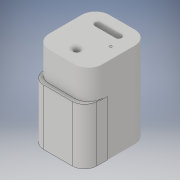
# Autodesk Inventor part: pencil sharpener
Saved by Autodesk Inventor 2017 (Build 210142000, 142)
## iProperties
Created: 2018-03-27
Part Number: pencil sharpener
Material: Generic
Document SubType Name: Modeling
Designer: Braxton
Density: 1 g/cm^3
Appearance: Default
Author: Braxton
Autodesk Inventor part; units mm, degrees
ref_plane "YZ Plane" through (0, 0, 0) normal (1, 0, 0) x (0, 1, 0)
ref_plane "XZ Plane" through (0, 0, 0) normal (0, 1, 0) x (-1, 0, 0)
ref_plane "XY Plane" through (0, 0, 0) normal (0, 0, 1) x (1, 0, 0)
sketch "Sketch1" plane through (0, 0, 0) normal (0, 1, 0) x (-1, 0, 0)
  line L0 (4.0465, 0) -> (4.0465, -4.1391)
  line L1 (1.9447, -6.241) -> (0, -6.241)
  arc A0 (1.9447, -6.241) -> (4.0465, -4.1391) centre (1.9447, -4.1391) ccw
  line L2 (4.0465, 0) -> (0, 0)
  line L3 (0, 0) -> (0, -6.241) construction
  line L4 (-4.0465, 0) -> (-4.0465, -4.1391)
  line L5 (-1.9447, -6.241) -> (0, -6.241)
  arc A1 (-4.0465, -4.1391) -> (-1.9447, -6.241) centre (-1.9447, -4.1391) ccw
  line L6 (-4.0465, 0) -> (0, 0)
  line L7 (0, 0) -> (0, 2.7914) construction
  dimension "d9" = 6.241
  dimension "d11" = 4.0465
  dimension "d12" = 2.1019
  constraints: 16 end point, 4 point on circle, 3 symmetric about line, 2 centre point, 2 collinear, 2 horizontal, 2 perpendicular, 2 tangent, 2 vertical, 1 other
  measures "d9" distance between parallel lines of L2 L1
  measures "d11" distance between parallel lines of L0 L3
  measures "d12" radius of A0
extrude "bace bottom" add sketch "Sketch1" along normal blind 7.3163
sketch "Sketch3" plane through (0, 7.3163, 0) normal (0, 1, 0) x (1, 0, 0)
  line L0 (1.9447, 6.241) -> (-1.9447, 6.241) projected
  line L1 (0, 6.241) -> (0, -3.1186) construction
  line L2 (0, 6.241) -> (-1.9447, 6.241)
  arc A0 (-1.9447, 6.241) -> (-4.0465, 4.1391) centre (-1.9447, 4.1391) ccw projected
  line L3 (-4.0465, 4.1391) -> (-4.0465, -0.825)
  line L4 (-1.9447, -2.9269) -> (0, -2.9269)
  arc A1 (-4.0465, -0.825) -> (-1.9447, -2.9269) centre (-1.9447, -0.825) ccw
  arc A2 (-1.9447, 6.241) -> (-4.0465, 4.1391) centre (-1.9447, 4.1391) ccw
  line L5 (0, 6.241) -> (1.9447, 6.241)
  arc A3 (4.0465, 4.1391) -> (1.9447, 6.241) centre (1.9447, 4.1391) ccw
  line L6 (4.0465, 4.1391) -> (4.0465, -0.825)
  line L7 (1.9447, -2.9269) -> (0, -2.9269)
  arc A4 (1.9447, -2.9269) -> (4.0465, -0.825) centre (1.9447, -0.825) ccw
  constraints: 14 end point, 8 point on circle, 5 symmetric about line, 5 tangent, 4 centre point, 2 vertical, 1 equal radius, 1 horizontal, 1 midpoint, 1 perpendicular, 1 point on line, 2 other
extrude "sharpener top" add sketch "Sketch3" along normal blind 4.6207
sketch "Sketch6" plane through (0, 0, 0) normal (1, 0, 0) x (0, 1, 0)
  line L0 (11.9369, 0.825) -> (11.9369, 2.9269) projected
  arc A0 (11.2464, 0.9441) -> (11.9369, 1.6347) centre (11.2464, 1.6347) ccw
  arc A1 (11.9369, -0.3815) -> (11.2464, 0.3091) centre (11.2464, -0.3815) ccw construction
  line L1 (11.9369, -4.1391) -> (11.9369, 0.825) projected
  line L2 (11.2464, 0.6266) -> (11.9369, 0.6266)
  line L3 (11.2464, 0.9441) -> (11.2464, 0.6266)
  line L4 (11.2464, 0.3091) -> (11.2464, 0.6266) construction
  line L5 (11.9369, 1.6347) -> (11.9369, 0.6266)
  line L6 (7.3163, 2.9269) -> (11.9369, 2.9269) projected
  point P0 (0, 0)
  dimension "d34" = 1.2922
  dimension "d37" = 2.0161
  constraints: 8 end point, 4 point on circle, 3 collinear, 3 point on line, 3 tangent, 2 centre point, 2 line through centre, 1 equal radius, 1 perpendicular, 1 vertical
  measures "d34" distance from line of L5.start L6
  measures "d37" distance of A1.start L5.start
revolve "sharpener hole" cut sketch "Sketch6" angle 360 about axis through (0, 11.2464, 0.6266) along (0, 1, 0)
sketch "Sketch7" plane through (0, 11.2464, 0.6266) normal (0, 1, 0) x (1, 0, 0)
  circle A0 centre (0, 0) radius 0.3175 projected
  circle A1 centre (0, 0) radius 0.3897
  point P0 (0, 0.6266)
  constraints: 1 centre point, 1 coincident
extrude "Extrusion of sharpener hole" cut sketch "Sketch7" against normal blind 1.5875 contours A0
sketch "Sketch8" plane through (0, 11.9369, 0) normal (0, 1, 0) x (1, 0, 0)
  line L0 (-1.5785, 4.1397) -> (1.5785, 4.1397) construction
  line L1 (-1.5785, 3.6661) -> (1.5785, 3.6661)
  line L2 (1.5785, 4.6133) -> (-1.5785, 4.6133)
  arc A0 (-1.5785, 4.6133) -> (-1.5785, 3.6661) centre (-1.5785, 4.1397) ccw
  arc A1 (1.5785, 3.6661) -> (1.5785, 4.6133) centre (1.5785, 4.1397) ccw
  line L3 (0, 4.6133) -> (0, 3.6661) construction
  line L4 (1.9447, 6.241) -> (-1.9447, 6.241) projected
  line L5 (0, 6.241) -> (0, 6.8422) construction
  point P0 (0, 0)
  point P1 (0, 4.1397)
  point P2 (-2.0521, 4.1397)
  point P3 (2.0521, 4.1397)
  dimension "d44" = 1.6277
  dimension "d45" = 0.9472
  dimension "d47" = 4.1042
  constraints: 12 end point, 6 point on circle, 4 midpoint, 4 tangent, 2 centre point, 1 collinear, 1 horizontal, 1 parallel, 1 perpendicular, 1 vertical
  measures "d44" distance between parallel lines of L4 L2
  measures "d45" distance between parallel lines of L2 L1
  measures "d47" distance of point (2.052, 4.14) point (-2.052, 4.14)
extrude "pencil holder" cut sketch "Sketch8" against normal blind 1.3843
sketch "Sketch9" plane through (0, 10.5526, 0) normal (0, 1, 0) x (1, 0, 0)
  line L0 (-0.0534, 4.6133) -> (-0.0534, 3.6661)
  line L1 (0, 3.5898) -> (0, 4.7623) construction
  line L2 (0.0534, 4.6133) -> (0.0534, 3.6661)
  line L3 (0, 0) -> (0, 2.9874)
  line L4 (-1.9447, 6.241) -> (1.9447, 6.241) projected
  line L5 (-1.5785, 4.6133) -> (1.5785, 4.6133) projected
  line L6 (-0.0534, 4.6133) -> (-1.5785, 4.6133)
  line L7 (1.5785, 3.6661) -> (-1.5785, 3.6661) projected
  line L8 (-0.0534, 3.6661) -> (-1.5785, 3.6661)
  arc A0 (1.5785, 3.6661) -> (1.5785, 4.6133) centre (1.5785, 4.1397) ccw projected
  line L9 (1.5785, 3.6661) -> (0.0534, 3.6661)
  line L10 (0.0534, 4.6133) -> (1.5785, 4.6133)
  arc A1 (-1.5785, 4.6133) -> (-1.5785, 3.6661) centre (-1.5785, 4.1397) ccw projected
  arc A2 (-1.5785, 4.6133) -> (-1.5785, 4.6133) centre (-1.5785, 4.1397) ccw
  arc A3 (-1.5785, 4.6133) -> (-1.5785, 3.6661) centre (-1.5785, 4.1397) ccw
  arc A4 (1.5785, 3.6661) -> (1.5785, 4.6133) centre (1.5785, 4.1397) ccw
  dimension "d39" = 0.1069
  constraints: 16 end point, 5 tangent, 4 point on circle, 3 collinear, 2 centre point, 2 horizontal, 2 symmetric about line, 1 point on line, 1 vertical, 1 vertical alignment, 3 other
  measures "d39" distance between parallel lines of L2 L0
extrude "pencil holder bottom" cut sketch "Sketch9" against normal blind 1.5875 contours L0 L7 A2 L5 | A2 A1 | L5 A0 L7 L2
sketch "Sketch12" plane through (0, 11.9369, 0) normal (0, 1, 0) x (1, 0, 0)
  circle A0 centre (2.3273, 2.186) radius 0.1969
  arc A1 (1.5785, 3.6661) -> (1.5785, 4.6133) centre (1.5785, 4.1397) ccw projected
  point P0 (0, 0)
  point P1 (2.0521, 4.1397)
  dimension "d48" = 0.3937
  dimension "d50" = 1.9537
  dimension "d51" = 0.2752
  constraints: 2 point on circle, 1 centre point
  measures "d48" diameter of A0
  measures "d50" vertical distance of point (2.052, 4.14) A0.centre
  measures "d51" horizontal distance of A0.centre point (2.052, 4.14)
extrude "sharpened light hole" cut sketch "Sketch12" against normal blind 1.5875
sketch "Sketch13" plane through (2.3273, 10.3494, -2.186) normal (0, 1, 0) x (1, 0, 0)
  circle A0 centre (0, 0) radius 0.1609
  point P0 (-2.3273, -2.186)
  dimension "d54" = 0.3217
  constraints: 1 centre point
  measures "d54" diameter of A0
extrude "sharpened light indicator" add sketch "Sketch13" along normal up to surface (1.5875 mm away) separate body
sketch "Sketch10" plane through (0, 0, 0) normal (0, -1, 0) x (1, 0, 0)
  arc A0 (1.9447, -6.241) -> (4.0465, -4.1391) centre (1.9447, -4.1391) ccw projected
  arc A1 (-4.0465, -4.1391) -> (-1.9447, -6.241) centre (-1.9447, -4.1391) ccw projected
  line L0 (1.9447, -6.241) -> (-1.9447, -6.241)
  arc A2 (1.9447, -6.241) -> (4.0465, -4.1391) centre (1.9447, -4.1391) ccw
  arc A3 (-4.0465, -4.1391) -> (-1.9447, -6.241) centre (-1.9447, -4.1391) ccw
  arc A4 (-1.9447, 2.7216) -> (-3.8412, 0.825) centre (-1.9447, 0.825) ccw
  line L1 (-1.9447, 2.7216) -> (1.9447, 2.7216)
  arc A5 (3.8412, 0.825) -> (1.9447, 2.7216) centre (1.9447, 0.825) ccw
  line L2 (-3.8412, 0.825) -> (-3.8412, 0)
  line L3 (4.0465, 0) -> (-4.0465, 0) projected
  line L4 (3.8412, 0.825) -> (3.8412, 0)
  line L5 (-4.0465, 0.825) -> (-3.8412, 0.825) construction
  line L6 (4.0465, 0.825) -> (4.0465, -4.1391) projected
  line L7 (4.0465, 0.825) -> (3.8412, 0.825) construction
  line L8 (-3.6719, 0) -> (-3.6719, 0.825)
  arc A6 (-1.9447, 2.5522) -> (-3.6719, 0.825) centre (-1.9447, 0.825) ccw
  line L9 (-1.9447, 2.5522) -> (1.9447, 2.5522)
  arc A7 (3.6719, 0.825) -> (1.9447, 2.5522) centre (1.9447, 0.825) ccw
  line L10 (3.6719, 0.825) -> (3.6719, 0)
  line L11 (3.8412, 0) -> (4.0465, 0)
  line L12 (4.0465, 0) -> (4.0465, -4.1391)
  line L13 (-4.0465, -4.1391) -> (-4.0465, 0)
  line L14 (-3.8412, 0) -> (-4.0465, 0)
  line L15 (-3.6719, 0) -> (3.6719, 0)
  point P0 (1.9447, 2.9269)
  point P1 (-1.9447, 2.9269)
  dimension "d29" = 0.2053
  dimension "d30" = 0.2053
  dimension "d31" = 0.2053
  dimension "d32" = 0.2053
  dimension "d33" = 0.1693
  constraints: 28 end point, 12 point on circle, 6 centre point, 6 tangent, 3 horizontal, 3 parallel, 2 collinear, 2 perpendicular, 2 point on line, 1 concentric, 1 vertical, 4 other
  measures "d29" distance of L6.start L4.start
  measures "d30" distance of L5.start L2.start
  measures "d31" distance from line of L1 point (1.945, 2.927)
  measures "d32" distance of L1.start point (-1.945, 2.927)
  measures "d33" distance between parallel lines of L1 L9
extrude "bottom of bace" add sketch "Sketch10" along normal blind 1.0372 contours L0 A1 L13 L3 L6 A0 | L3 L10 A7 L9 A6 L8 L2 A4 L1 A5 L4 bodies 1
sketch "Sketch14" plane through (-1.9447, 0, 2.7216) normal (0, 0, 1) x (1, 0, 0)
  line L0 (1.9447, 0) -> (1.6071, 0)
  line L1 (1.6071, 0) -> (1.6071, -0.6763)
  line L2 (1.9447, 0) -> (2.2823, 0)
  line L3 (2.2823, -0.6763) -> (2.2823, 0)
  line L4 (2.2823, -0.6763) -> (1.6071, -0.6763)
  dimension "d57" = 0.3376
  dimension "d59" = 0.6763
  dimension "d60" = 0.3376
  constraints: 10 end point, 2 perpendicular, 1 vertical
  measures "d57" distance of L0.start L0.end
  measures "d59" distance of L0.end L1.end
  measures "d60" distance of L0.start L2.end
extrude "cut for holder" cut sketch "Sketch14" against normal up to surface (0.1693 mm away) bodies 1
sketch "Sketch11" plane through (0, -1.0372, 0) normal (0, -1, 0) x (1, 0, 0)
  line L0 (3.6719, 0.825) -> (3.6719, 0) projected
  line L1 (3.6719, 0) -> (3.6719, 0.825)
  arc A0 (3.6719, 0.825) -> (1.9447, 2.5522) centre (1.9447, 0.825) ccw projected
  arc A1 (-1.9447, 2.5522) -> (-3.6719, 0.825) centre (-1.9447, 0.825) ccw projected
  line L2 (1.9447, 2.5522) -> (-1.9447, 2.5522) projected
  line L3 (-1.9447, 2.5522) -> (1.9447, 2.5522)
  line L4 (-3.6719, 0.825) -> (-3.6719, 0) projected
  line L5 (-3.6719, 0) -> (-3.6719, 0.825)
  line L6 (3.6719, 0) -> (-3.6719, 0)
  line L7 (-1.9447, 2.5522) -> (1.9447, 2.5522) projected
  arc A2 (-1.9447, 2.5522) -> (-3.6719, 0.825) centre (-1.9447, 0.825) ccw
  arc A3 (3.6719, 0.825) -> (1.9447, 2.5522) centre (1.9447, 0.825) ccw
  point P0 (0, 0)
  constraints: 8 end point, 4 point on circle, 3 collinear, 2 centre point, 2 concentric, 1 horizontal
extrude "bottom of tray slot" add sketch "Sketch11" against normal blind 0.2043 bodies 1
sketch "Sketch15" plane through (0, -1.0372, 0) normal (0, -1, 0) x (1, 0, 0)
  line L0 (-4.0465, 0) -> (-4.0465, 1.6234)
  line L1 (4.0465, 0.825) -> (4.0465, 0) projected
  line L2 (4.0465, 0) -> (4.0465, 1.6234)
  arc A0 (4.0465, 1.6234) -> (2.15, 3.5199) centre (2.15, 1.6234) ccw
  arc A1 (-2.15, 3.5199) -> (-4.0465, 1.6234) centre (-2.15, 1.6234) ccw
  line L3 (-2.15, 3.5199) -> (2.15, 3.5199)
  line L4 (3.8412, 0) -> (3.6719, 0) projected
  line L5 (3.8412, 0.825) -> (3.8412, 1.6234)
  line L6 (-3.8412, 0.825) -> (-3.8412, 1.6234)
  line L7 (-3.8412, 0) -> (-4.0465, 0) projected
  line L8 (-3.8412, 0) -> (-4.0465, 0)
  line L9 (3.8412, 0) -> (4.0465, 0)
  line L10 (4.0465, 0.825) -> (4.0465, -4.1391) projected
  arc A2 (3.8412, 1.6234) -> (2.15, 3.3146) centre (2.15, 1.6234) ccw
  arc A3 (-2.15, 3.3146) -> (-3.8412, 1.6234) centre (-2.15, 1.6234) ccw
  line L11 (2.15, 3.3146) -> (-2.15, 3.3146)
  arc A4 (-1.9447, 2.7216) -> (-3.8412, 0.825) centre (-1.9447, 0.825) ccw projected
  arc A5 (3.8412, 0.825) -> (1.9447, 2.7216) centre (1.9447, 0.825) ccw projected
  arc A6 (3.8412, 0.825) -> (1.9447, 2.7216) centre (1.9447, 0.825) ccw
  line L12 (1.9447, 2.7216) -> (-1.9447, 2.7216) projected
  line L13 (-3.8412, 0.825) -> (-3.8412, 0) projected
  arc A7 (-1.9447, 2.7216) -> (-3.8412, 0.825) centre (-1.9447, 0.825) ccw
  line L14 (-1.9447, 2.7216) -> (1.9447, 2.7216)
  line L15 (1.9447, 2.5522) -> (-1.9447, 2.5522) projected
  line L16 (3.8412, 0.825) -> (3.8412, 0)
  line L17 (-3.8412, 0.825) -> (-3.8412, 0)
  point P0 (0, 0)
  constraints: 22 end point, 14 point on circle, 8 tangent, 6 centre point, 5 vertical, 3 concentric, 3 parallel, 2 equal radius, 2 horizontal, 1 perpendicular
sketch "Sketch16" plane through (-0.3376, -0.6763, 2.7216) normal (0, 1, 0) x (1, 0, 0)
  line L0 (0, 0) -> (0, 0.4561)
  line L1 (0, 0.4561) -> (0.1312, 0.4561)
  line L2 (0.1312, 0.4561) -> (0.1312, 0)
  line L3 (0.1312, 0) -> (0, 0)
  line L4 (0.6752, 0.1693) -> (0.6752, 0) projected
  line L5 (0.6752, 0) -> (0.6752, 0.4561)
  line L6 (0.6752, 0.4561) -> (0.544, 0.4561)
  line L7 (0.544, 0.4561) -> (0.544, 0)
  line L8 (0.6752, 0) -> (0, 0) projected
  line L9 (0.6752, 0) -> (0.544, 0)
  point P0 (0.3376, 2.7216)
  dimension "d68" = 0.4561
  dimension "d69" = 0.1312
  constraints: 16 end point, 5 perpendicular, 2 collinear, 2 equal length, 1 point on line, 1 vertical
  measures "d68" distance of L0.start L0.end
  measures "d69" distance of L0.end L1.end
extrude "nobes for connection" add sketch "Sketch16" along normal up to surface (0.6763 mm away) bodies 1
extrude "connection to nobes" add sketch "Sketch15" against normal up to surface (1.0372 mm away) contours L6 A3 L11 A2 L5 A5 L12 A4 bodies 1
sketch "Sketch18" plane through (0, 0, 0) normal (0, 1, 0) x (1, 0, 0)
  line L0 (-3.8412, -1.6234) -> (-3.8412, 0) projected
  line L1 (-3.8412, 0) -> (-3.8412, -1.6234)
  arc A0 (-3.8412, -1.6234) -> (-2.15, -3.3146) centre (-2.15, -1.6234) ccw projected
  arc A1 (2.15, -3.3146) -> (3.8412, -1.6234) centre (2.15, -1.6234) ccw projected
  line L2 (2.15, -3.3146) -> (-2.15, -3.3146) projected
  line L3 (2.15, -3.3146) -> (-2.15, -3.3146)
  line L4 (3.8412, 0) -> (3.8412, -1.6234) projected
  line L5 (3.8412, -1.6234) -> (3.8412, 0)
  line L6 (-3.6719, 0) -> (3.6719, 0) projected
  line L7 (-3.8412, 0) -> (-2.9543, 0)
  line L8 (-2.9543, 0) -> (-2.9543, -0.798)
  line L9 (-2.9543, -0.798) -> (-1.6272, -0.798)
  line L10 (3.8412, 0) -> (2.9543, 0)
  line L11 (2.9543, 0) -> (2.9543, -0.798)
  line L12 (2.9543, -0.798) -> (1.6272, -0.798)
  line L13 (-0.2064, -2.5522) -> (-0.2064, -2.2654) projected
  line L14 (0.3376, -2.2654) -> (0.2064, -2.2654) projected
  line L15 (-0.2064, -2.2654) -> (0.2064, -2.2654)
  arc A2 (-1.6272, -0.798) -> (1.6272, -0.798) centre (0, -0.5193) ccw
  point P0 (0, 0)
  point P1 (-3.6719, -0.825)
  point P2 (0, -2.1702)
  dimension "d76" = 0.8869
  dimension "d77" = 0.798
  dimension "d78" = 1.3272
  dimension "d79" = 0.0953
  constraints: 20 end point, 3 equal length, 3 horizontal, 3 point on circle, 2 collinear, 2 point on line, 2 vertical, 1 centre point, 1 parallel
  measures "d76" distance of L0.end L7.end
  measures "d77" distance of L7.end L8.end
  measures "d78" distance of L8.end L9.end
  measures "d79" distance from line of point (0, -2.17) L15
extrude "holding slot bottom" add sketch "Sketch18" along normal blind 0.163 contours L0 L7 L6 L8 L9 A2 L12 L11 L10 L4 A1 L2 A0 bodies 1
sketch "Sketch19" plane through (0, 0.163, 0) normal (0, 1, 0) x (1, 0, 0)
  line L0 (2.9543, 0) -> (2.9543, -0.798) projected
  line L1 (2.9543, 0) -> (2.9543, -0.798)
  arc A0 (-1.6272, -0.798) -> (1.6272, -0.798) centre (0, -0.5193) ccw projected
  line L2 (2.9543, -0.798) -> (1.6272, -0.798)
  line L3 (-2.9543, 0) -> (-2.9543, -0.798)
  line L4 (-2.9543, -0.798) -> (-1.6272, -0.798)
  line L5 (3.8412, -0.1566) -> (3.111, -0.1566)
  line L6 (3.111, -0.1566) -> (3.111, -0.9546)
  line L7 (3.111, -0.9546) -> (1.7543, -0.9546)
  arc A1 (-1.6272, -0.798) -> (1.6272, -0.798) centre (0, -0.5193) ccw
  arc A2 (-1.7543, -0.9546) -> (1.7543, -0.9546) centre (0, -0.5193) ccw
  line L8 (-3.8412, -0.1566) -> (-3.111, -0.1566)
  line L9 (-3.111, -0.1566) -> (-3.111, -0.9546)
  line L10 (-3.111, -0.9546) -> (-1.7543, -0.9546)
  line L11 (3.8412, 0) -> (3.8412, -1.6234) projected
  line L12 (3.8412, 0) -> (3.8412, -0.1566)
  line L13 (-3.8412, -1.6234) -> (-3.8412, 0) projected
  line L14 (-2.9543, 0) -> (-3.6719, 0) projected
  line L15 (-3.8412, 0) -> (-2.9543, 0)
  line L16 (-3.8412, -0.1566) -> (-3.8412, 0)
  line L17 (2.9543, 0) -> (3.8412, 0)
  line L18 (-3.6719, 0) -> (3.6719, 0) projected
  point P0 (0, 0)
  dimension "d86" = 0.1566
  dimension "d87" = 0.1566
  dimension "d88" = 0.1566
  dimension "d89" = 0.1566
  constraints: 28 end point, 7 perpendicular, 5 point on circle, 4 collinear, 3 equal length, 2 centre point, 2 concentric, 2 horizontal, 2 point on line
  measures "d86" distance of L11.start L5.start
  measures "d87" distance between parallel lines of L0 L6
  measures "d88" distance between parallel lines of L2 L7
  measures "d89" radial gap between concentric circles of A0 A2
extrude "holding slot back" add sketch "Sketch19" along normal blind 5.2102 contours L17 L11 L5 L6 L7 A2 L10 L9 L8 L13 L15 L14 L3 L4 A0 L2 L0 bodies 1
sketch "Sketch20" plane through (-3.111, 0.163, 0.9546) normal (0, 0, 1) x (1, 0, 0)
  line L0 (1.4838, 5.2102) -> (4.7382, 5.2102) projected
  line L1 (3.111, 5.2102) -> (3.111, 4.5551) construction
  line L2 (3.111, 4.5551) -> (2.4723, 4.5551)
  line L3 (2.4723, 4.5551) -> (2.4723, 5.2102)
  line L4 (2.4723, 5.2102) -> (3.111, 5.2102)
  line L5 (3.111, 4.5551) -> (3.7497, 4.5551)
  line L6 (3.7497, 4.5551) -> (3.7497, 5.2102)
  line L7 (3.7497, 5.2102) -> (3.111, 5.2102)
  point P0 (3.111, -0.163)
  dimension "d92" = 0.6551
  dimension "d93" = 0.6387
  constraints: 14 end point, 2 perpendicular, 2 symmetric about line, 1 collinear, 1 midpoint, 1 point on line, 1 vertical
  measures "d92" distance of L1.start L1.end
  measures "d93" distance of L1.end L2.end
extrude "holding slot back cut" cut sketch "Sketch20" along normal up to surface bodies 1
extrude "container for wasts" add sketch "Sketch15" against normal up to surface (8.3534 mm away) separate body contours L0 A1 L3 A0 L2 L1 L9 L16 L5 A2 L11 A3 L6 L13 L7
sketch "Sketch21" plane through (-2.15, 7.3163, 3.3146) normal (0, 1, 0) x (1, 0, 0)
  arc A0 (-1.8965, 2.4895) -> (0.2053, 0.3877) centre (0.2053, 2.4895) ccw projected
  line L0 (0.2053, 0.3877) -> (4.0947, 0.3877) projected
  arc A1 (-1.8965, 2.4895) -> (0.2053, 0.3877) centre (0.2053, 2.4895) ccw
  arc A2 (4.0947, 0.3877) -> (6.1965, 2.4895) centre (4.0947, 2.4895) ccw projected
  arc A3 (4.0947, 0.3877) -> (6.1965, 2.4895) centre (4.0947, 2.4895) ccw
  line L1 (0, -0.2053) -> (4.3, -0.2053) projected
  arc A4 (4.3, -0.2053) -> (6.1965, 1.6912) centre (4.3, 1.6912) ccw projected
  arc A5 (4.3, -0.2053) -> (4.3, -0.2053) centre (4.3, 1.6912) ccw
  line L2 (-1.8965, 1.6912) -> (-1.8965, 3.3146) projected
  arc A6 (-1.8965, 1.6912) -> (0, -0.2053) centre (0, 1.6912) ccw projected
  arc A7 (-1.8965, 1.6912) -> (-1.8965, 1.6912) centre (0, 1.6912) ccw
  arc A8 (-1.8965, 1.6912) -> (0, -0.2053) centre (0, 1.6912) ccw
  line L3 (6.1965, 3.3146) -> (6.1965, 1.6912) projected
  arc A9 (4.3, -0.2053) -> (6.1965, 1.6912) centre (4.3, 1.6912) ccw
  line L4 (-1.8965, 1.6912) -> (-1.8965, 2.4895)
  line L5 (6.1965, 2.4895) -> (6.1965, 1.6912)
  line L6 (4.3, -0.2053) -> (0, -0.2053) projected
  line L7 (4.3, -0.2053) -> (0, -0.2053)
  line L8 (0.2053, 0.3877) -> (4.0947, 0.3877)
  point P0 (2.15, 3.3146)
  constraints: 8 end point, 8 point on circle, 8 tangent, 4 centre point, 3 concentric, 2 collinear, 1 horizontal, 1 horizontal alignment, 1 parallel, 1 vertical alignment, 7 other
extrude "holding area top" add sketch "Sketch21" along normal blind 0.1566 contours A0 A7 L2 | A0 L0 A7 A6 | A7 L0 A5 L1 | A5 L0 A2 A4 | A5 A2 L3 bodies 3
equation "\"d29\" = d32"
equation "\"d30\" = d32"
equation "\"d31\" = d32"
equation "\"d60\" = d57"
equation "\"d87\" = d86"
equation "\"d88\" = d86"
equation "\"d89\" = d86"
equation "\"d97\" = d86"
